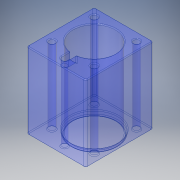
# Autodesk Inventor part: cylinder..
Saved by Autodesk Inventor 2017 (Build 210142000, 142)
## iProperties
Created: 2020-01-08
Part Number: cylinder..
Material: Stainless Steel
Document SubType Name: Modeling
Designer: Admin
Density: 8 g/cm^3
Appearance: Clear - Blue
Mass: 79.645 g
Surface Area: 58.9673 cm^2
Volume: 9.95563 cm^3
Author: Admin
Autodesk Inventor part; units mm, degrees
ref_plane "YZ Plane" through (0, 0, 0) normal (1, 0, 0) x (0, 1, 0)
ref_plane "XZ Plane" through (0, 0, 0) normal (0, 1, 0) x (-1, 0, 0)
ref_plane "XY Plane" through (0, 0, 0) normal (0, 0, 1) x (1, 0, 0)
sketch "Sketch1" plane through (0, 0, 0) normal (0, 1, 0) x (-1, 0, 0)
  line L0 (11.1125, -11.1125) -> (-11.1125, -11.1125)
  line L1 (-11.1125, -11.1125) -> (-11.1125, 14.2875)
  line L2 (-11.1125, 14.2875) -> (11.1125, 14.2875)
  line L3 (11.1125, 14.2875) -> (11.1125, -11.1125)
  point P0 (0, 0)
  dimension "d0" = 25.4
  dimension "d1" = 11.1125
  dimension "d2" = 11.1125
  dimension "d3" = 11.1125
  constraints: 8 end point, 2 parallel, 1 horizontal, 1 perpendicular
  measures "d0" distance of L2.end L0.start
  measures "d1" distance from line of L3 point (0, 0)
  measures "d2" distance from line of L1 point (0, 0)
  measures "d3" distance from line of point (0, 0) L0
extrude "Extrusion1" add sketch "Sketch1" against normal blind 30.1625
sketch "Sketch2" plane through (0, -30.1625, 0) normal (0, -1, 0) x (1, 0, 0)
  line L0 (-11.1125, 14.2875) -> (-11.1125, -11.1125) projected
  line L1 (11.1125, -11.1125) -> (11.1125, 14.2875) projected
  line L2 (-11.1125, -11.1125) -> (11.1125, -11.1125) projected
  point P0 (0, 0)
  point P1 (7.9375, -7.9375)
  point P2 (-7.9375, -7.9375)
  point P3 (-7.9375, 7.9375)
  point P4 (7.9375, 7.9375)
  dimension "d6" = 15.875
  dimension "d8" = 15.875
  dimension "d12" = 3.175
  dimension "d13" = 3.175
  dimension "d14" = 3.175
  dimension "d15" = 0
  dimension "d16" = 15.875
  dimension "d18" = 15.875
  measures "d6" distance of point (-7.938, -7.937) point (7.938, -7.938)
  measures "d8" distance of point (7.938, 7.938) point (-7.937, 7.938)
  measures "d12" distance from line of L1 point (7.938, 7.938)
  measures "d13" distance from line of L1 point (7.938, -7.938)
  measures "d14" distance from line of L2 point (7.938, -7.938)
  measures "d15" vertical distance of point (7.938, -7.938) point (-7.938, -7.937)
  measures "d16" distance of point (7.938, -7.938) point (7.938, 7.938)
  measures "d18" distance of point (-7.937, 7.938) point (-7.938, -7.937)
hole "Hole1" at (7.9375, -30.1625, -7.9375) at (-7.9375, -30.1625, -7.9375) at (-7.9375, -30.1625, 7.9375) at (7.9375, -30.1625, 7.9375) direction (0, 1, 0) diameter 2.2606 end through all
sketch "Sketch3" plane through (0, -30.1625, 0) normal (0, -1, 0) x (1, 0, 0)
  circle A0 centre (0, 0) radius 7.9375
  dimension "d26" = 15.875
  constraints: 1 centre point, 1 coincident
  measures "d26" diameter of A0
extrude "Extrusion2" cut sketch "Sketch3" against normal blind 30.1625
sketch "Sketch4" plane through (0, -30.1625, 0) normal (0, -1, 0) x (1, 0, 0)
  circle A0 centre (0, 0) radius 8.7313
  line L0 (-11.1125, -11.1125) -> (11.1125, -11.1125) projected
  line L1 (-11.1125, 14.2875) -> (-11.1125, -11.1125) projected
  line L2 (11.1125, -11.1125) -> (-11.1125, -11.1125)
  line L3 (-11.1125, -11.1125) -> (-11.1125, 14.2875)
  line L4 (-11.1125, 14.2875) -> (11.1125, 14.2875)
  line L5 (11.1125, 14.2875) -> (11.1125, -11.1125)
  dimension "d29" = 17.4625
  constraints: 8 end point, 2 parallel, 1 centre point, 1 coincident, 1 horizontal, 1 perpendicular
  measures "d29" diameter of A0
extrude "Extrusion3" cut sketch "Sketch4" against normal blind 1.5875
sketch "Sketch5" plane through (0, -28.575, 0) normal (0, -1, 0) x (1, 0, 0)
  point P0 (0, 0)
  point P1 (0, 11.1125)
  dimension "d32" = 11.1125
  dimension "d33" = 0
  measures "d32" distance of point (0, 0) point (0, 11.113)
  measures "d33" horizontal distance of point (0, 0) point (0, 11.113)
hole "Hole2" at (0, -28.575, 11.1125) direction (0, 1, 0) diameter 1.9837 end through all
sketch "Sketch6" plane through (0, 0, 0) normal (0, 1, 0) x (1, 0, 0)
  line L0 (-1.1906, -3.6864) -> (1.1906, -3.6864)
  line L1 (1.1906, -3.6864) -> (1.1906, -10.9137)
  line L2 (-1.1906, -10.9137) -> (-1.1906, -3.6864)
  circle A0 centre (0, -11.1125) radius 0.9922
  line L3 (-1.1906, -10.9137) -> (1.1906, -10.9137)
  arc A1 (-1.1906, -10.9137) -> (1.1906, -10.9137) centre (0, -10.9137) ccw
  circle A2 centre (0, -11.1125) radius 0.9919 projected
  point P0 (0, 0)
  dimension "d41" = 2.3813
  dimension "d42" = 1.1906
  dimension "d43" = 1.9844
  dimension "d44" = 0
  dimension "d45" = 11.1125
  dimension "d48" = 7.2273
  constraints: 8 end point, 3 tangent, 2 centre point, 2 horizontal, 2 point on circle, 1 parallel, 1 perpendicular
  measures "d41" distance between parallel lines of L1 L2
  measures "d42" distance from line of point (0, 0) L1
  measures "d43" diameter of A0
  measures "d44" horizontal distance of point (0, 0) A0.centre
  measures "d45" distance of A0.centre point (0, 0)
  measures "d48" distance between parallel lines of L3 L0
extrude "Extrusion4" cut sketch "Sketch6" against normal blind 2.3813
fillet "Fillet1" radius 0.7937 4 edges at (11.1125, -14.2875, -11.1125) (11.1125, -14.2875, 14.2875) (-11.1125, -14.2875, -11.1125) (-11.1125, -14.2875, 14.2875)
fillet "Fillet2" radius 0.3175 28 edges at (-8.7313, -28.575, 0) (-7.9375, -30.1625, 0) (-8.7313, -30.1625, 0) (7.9375, -28.575, -6.8072) (-7.9375, -28.575, -6.8072) (0, 0, -11.1125) (0, -28.575, -11.1125) (10.88, 0, -10.88) (11.1125, 0, 1.5875) (10.88, 0, 14.055) (0, 0, 14.2875) (-10.88, 0, 14.055) (-11.1125, 0, 1.5875) (-10.88, 0, -10.88) (-10.88, -28.575, -10.88) (-11.1125, -28.575, 1.5875) (-10.88, -28.575, 14.055) (0, -28.575, 14.2875) (10.88, -28.575, 14.055) (11.1125, -28.575, 1.5875) (10.88, -28.575, -10.88) (-7.9375, -28.575, 9.0678) (0, -28.575, 12.1044) (7.9375, -28.575, 9.0678) (-7.9375, 0, -6.8072) (-7.9375, 0, 9.0678) (7.9375, 0, 9.0678) (7.9375, 0, -6.8072)
fillet "Fillet3" radius 0.3175 8 edges at (-5.1746, 0, -6.0189) (6.0189, 0, 5.1746) (-1.1906, 0, 9.3807) (1.1906, 0, 9.3807) (0, 0, 12.1044) (0, -2.3813, 7.9375) (-1.1906, -1.1906, 7.8477) (1.1906, -1.1906, 7.8477)
body "Solid1"
